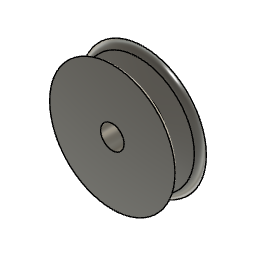
RoldanasBracosInferiores (Autodesk Fusion 360 design; units mm, degrees)
Autodesk Fusion 360 part; units mm, degrees
sketch "Esboço1" plane through (0, 0, 0) normal (0, 0, 1) x (1, 0, 0)
  line L0 (0, 0) -> (-40, 0)
  line L1 (0, 0) -> (0, 4.75)
  line L2 (0, 4.75) -> (-15, 4.75)
  line L3 (0, 20) -> (-40, 20)
  line L4 (0, 20) -> (0, 15.25)
  line L5 (0, 15.25) -> (-15, 15.25)
  line L6 (-15, 15.25) -> (-15, 4.75)
  line L7 (0, 15.25) -> (0, 4.75)
  line L8 (-40, 0) -> (-40, 3)
  line L9 (-40, 20) -> (-40, 17)
  line L10 (-40, 17) -> (-15, 15.25)
  line L11 (-40, 3) -> (-15, 4.75)
  constraint coincident L0.start L1.start
  constraint horizontal L0
  constraint perpendicular L0 L1
  constraint perpendicular L1 L2
  constraint parallel L0 L3
  constraint perpendicular L3 L4
  constraint perpendicular L4 L5
  constraint perpendicular L2 L6
  constraint perpendicular L2 L7
  constraint perpendicular L0 L8
  constraint perpendicular L3 L9
revolve "Revolucionar1" add sketch "Esboço1" angle 360 about axis through (0, 15.25, 0) along (0, -1, 0)
fillet "Arredondamento1" radius 5 2 faces at (12.584, 16.6111, 32.0634) (-7.6646, 3.3889, 33.5809)
hole "Furo1" at (0, 20, 0) direction (0, -1, 0) diameter 15 depth 30 tip angle 118
